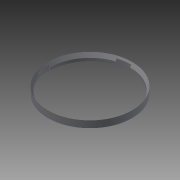
# Autodesk Inventor part: diffuser75
Saved by Autodesk Inventor 2014 (Build 180170000, 170)
## iProperties
Created: 2014-07-05
Part Number: diffuser75
Material: Generic
Document SubType Name: Modeling
Designer: lukeiseman
Density: 1 g/cm^3
Appearance: Default
Author: lukeiseman
Autodesk Inventor part; units mm, degrees
ref_plane "YZ Plane" through (0, 0, 0) normal (1, 0, 0) x (0, 1, 0)
ref_plane "XZ Plane" through (0, 0, 0) normal (0, 1, 0) x (-1, 0, 0)
ref_plane "XY Plane" through (0, 0, 0) normal (0, 0, 1) x (1, 0, 0)
sketch "Sketch1" plane through (0, 0, 0) normal (0, 1, 0) x (-1, 0, 0)
  circle A0 centre (0, 0) radius 47.625
  circle A1 centre (0, 0) radius 45.5168
  dimension "d0" = 95.25
  dimension "d1" = 91.0336
  constraints: 2 centre point, 2 coincident
  measures "d0" diameter of A0
  measures "d1" diameter of A1
sketch "Sketch2" plane through (0, 0, 0) normal (1, 0, 0) x (0, 1, 0)
  line L0 (0, -47.625) -> (0, 47.625) projected
  line L1 (0, -45.5168) -> (0, 45.5168) projected
  line L2 (0, 0) -> (0, -45.5168)
  line L3 (15.24, -45.5168) -> (0, -45.5168)
  line L4 (0, -47.625) -> (32.7797, -47.625)
  line L5 (7.62, -47.625) -> (3.175, -45.5168)
  line L6 (-6.5559, 0) -> (39.3357, 0) projected
  constraints: 8 end point, 2 point on line, 1 collinear, 1 parallel, 1 perpendicular
revolve "Revolution1" add sketch "Sketch2" angle 360 about axis through (0, -10, 0) along (0, 1, 0)
sketch "Sketch3" plane through (0, 0, 0) normal (0, 1, 0) x (-1, 0, 0)
  circle A0 centre (0, 0) radius 43.8086
  line L0 (0, 43.8086) -> (0, 46.5836)
  line L1 (41.6644, 13.5376) -> (44.3036, 14.3951)
  line L2 (43.8086, 0) -> (46.5836, 0) construction
  line L3 (0, 0) -> (46.5836, 0)
  line L4 (-13.5376, 41.6644) -> (-14.3951, 44.3036)
  line L5 (0, 0) -> (46.5836, 0) construction
  line L6 (-43.8086, 0) -> (-46.5836, 0)
  line L7 (-41.6644, -13.5376) -> (-44.3036, -14.3951)
  line L8 (0, 0) -> (46.5836, 0) construction
  line L9 (0, -43.8086) -> (0, -46.5836)
  line L10 (13.5376, -41.6644) -> (14.3951, -44.3036)
  line L11 (0, 0) -> (46.5836, 0) construction
  arc A1 (0, 46.5836) -> (-14.3951, 44.3036) centre (0, 0) ccw
  arc A2 (-46.5836, 0) -> (-44.3036, -14.3951) centre (0, 0) ccw
  arc A3 (0, -46.5836) -> (14.3951, -44.3036) centre (0, 0) ccw
  arc A4 (46.5836, 0) -> (44.3036, 14.3951) centre (0, 0) ccw
  arc A5 (0, -43.8086) -> (13.5376, -41.6644) centre (0, 0) ccw
  arc A6 (-43.8086, 0) -> (-41.6644, -13.5376) centre (0, 0) ccw
  arc A7 (43.8086, 0) -> (41.6644, 13.5376) centre (0, 0) ccw
  arc A8 (0, 43.8086) -> (-13.5376, 41.6644) centre (0, 0) ccw
  line L12 (46.5836, 0) -> (43.8086, 0)
  dimension "d5" = 18
  dimension "d6" = 108
  dimension "d7" = 162
  dimension "d8" = 72
  constraints: 26 end point, 16 point on circle, 8 centre point, 8 coincident, 4 horizontal, 4 perpendicular, 3 collinear, 1 vertical, 10 other
  measures "d5" angle of L2 L1
  measures "d6" angle of L5 L4
  measures "d7" angle of L7 L8
  measures "d8" angle of L10 L11
extrude "Extrusion1" cut sketch "Sketch3" along normal blind 25.4 contours A0 L1 A4 L3 | L10 A3 L9 A0 | A0 L4 A1 L0 | L7 A2 L6 A0
body "Solid1"
